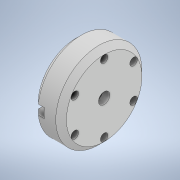
# Autodesk Inventor part: 711134
Saved by Autodesk Inventor 2022 (Build 260153000, 153)
## iProperties
Created: 2021-10-22
Part Number: 711134
Material: Типовые
Document SubType Name: Modeling
Designer: RaNSiD
Density: 1 g/cm^3
Appearance: По умолчанию
Mass: 20.8625 g
Surface Area: 65.1231 cm^2
Volume: 20.8625 cm^3
Author: RaNSiD
Autodesk Inventor part; units mm, degrees
ref_plane "YZ Plane" through (0, 0, 0) normal (1, 0, 0) x (0, 1, 0)
ref_plane "XZ Plane" through (0, 0, 0) normal (0, 1, 0) x (-1, 0, 0)
ref_plane "XY Plane" through (0, 0, 0) normal (0, 0, 1) x (1, 0, 0)
sketch "Эскиз1" plane through (-7.5, -11.4142, 0) normal (0, 0, 1) x (1, 0, 0)
  line L0 (0, 0) -> (0, 20)
  line L1 (0, 20) -> (2.8284, 22.8284)
  line L2 (0, 0) -> (15, 0)
  line L3 (15, 0) -> (15, 20)
  line L4 (15, 20) -> (12.1716, 22.8284)
  line L5 (12.1716, 22.8284) -> (2.8284, 22.8284)
  dimension "d5" = 20
  dimension "d4" = 4
  dimension "d3" = 135
  dimension "d2" = 15
  dimension "d1" = 4
  dimension "d0" = 135
  constraints: 12 end point, 1 horizontal, 1 parallel, 1 perpendicular, 1 vertical
  measures "d5" distance of L0.start L0.end
  measures "d4" distance of L0.end L1.end
  measures "d3" angle of L0 L1
  measures "d2" distance of L0.start L2.end
  measures "d1" distance of L3.end L4.end
  measures "d0" angle of L4 L3
revolve "Вращение1" add sketch "Эскиз1" angle 360 about axis through (-7.5, -11.4142, 0) along (1, 0, 0)
sketch "Эскиз2" plane through (0, 0, 0) normal (0, 0, 1) x (1, 0, 0)
  line L0 (7.5, -8.4142) -> (3.7, -8.4142)
  line L1 (7.5, -11.4142) -> (7.5, -8.4142)
  line L2 (3.7, -7.7142) -> (3, -7.7142)
  line L3 (3, -7.7142) -> (3, -11.4142)
  line L4 (3, -11.4142) -> (7.5, -11.4142)
  line L5 (3.7, -8.4142) -> (3.7, -7.7142)
  line L6 (7.5, -31.4142) -> (7.5, 8.5858) projected
  point P0 (0, 0)
  dimension "d7" = 4.5
  dimension "d8" = 0.7
  dimension "d10" = 3
  dimension "d9" = 0.7
  dimension "d26" = 11.4142
  constraints: 12 end point, 2 horizontal, 2 parallel, 1 midpoint, 1 perpendicular
  measures "d7" distance between parallel lines of L3 L1
  measures "d8" distance of L2.start L2.end
  measures "d10" distance of L1.start L0.start
  measures "d9" distance of L0.end L2.start
  measures "d26" vertical distance of point (0, 0) L1.start
revolve "Вращение2" cut sketch "Эскиз2" angle 360 about axis through (3, -11.4142, 0) along (1, 0, 0)
sketch "Эскиз3" plane through (7.5, -11.4142, 0) normal (1, 0, 0) x (0, 0, -1)
  circle A0 centre (0, 0) radius 3 construction
  point P0 (0, 11.4142)
  point P1 (0, 18)
  point P2 (-15.5885, 9)
  point P3 (-15.5885, -9)
  point P4 (0, -18)
  point P5 (15.5885, -9)
  point P6 (15.5885, 9)
  dimension "d14" = 18
  dimension "d17" = 360
  constraints: 1 vertical alignment, 7 other
  measures "d14" distance of point (0, 18) A0.centre
hole "Отверстие1" at (7.5, 6.5858, 0) at (7.5, -2.4142, 15.5885) at (7.5, -20.4142, 15.5885) at (7.5, -29.4142, 0) at (7.5, -20.4142, -15.5885) at (7.5, -2.4142, -15.5885) direction (-1, 0, 0) diameter 4 end through all
sketch "Эскиз4" plane through (0, 0, 0) normal (0, 0, 1) x (1, 0, 0)
  line L0 (-7.5, -21.4142) -> (-7.5, -1.4142) construction
  line L1 (-1.5, -8.9142) -> (-7.5, -8.9142)
  line L2 (-7.5, -8.9142) -> (-7.5, -13.9142)
  line L3 (-7.5, -13.9142) -> (-1.5, -13.9142)
  line L4 (-1.5, -13.9142) -> (-1.5, -8.9142)
  line L5 (7.5, -21.4142) -> (7.5, -1.4142) construction
  point P0 (0, 0)
  point P1 (-7.5, -11.4142)
  point P2 (7.5, -11.4142)
  dimension "d27" = 5
  dimension "d28" = 6
  constraints: 8 end point, 2 midpoint, 2 parallel, 1 horizontal, 1 horizontal alignment, 1 perpendicular, 1 point on line
  measures "d27" distance of L3.end L1.start
  measures "d28" distance of L1.start L1.end
extrude "Выдавливание1" cut sketch "Эскиз4" along normal through all both and the other way through all
